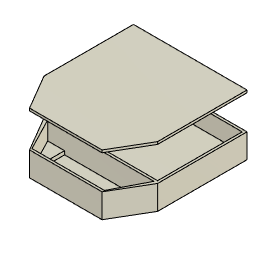
mainboard v1 (Autodesk Fusion 360 design; units mm, degrees)
Autodesk Fusion 360 part; units mm, degrees
sketch "Sketch1" plane through (0, 0, 0) normal (0, 0, 1) x (1, 0, 0)
  line L0 (0, 0) -> (90, 0)
  line L1 (90, 0) -> (90, 70)
  line L2 (90, 70) -> (0, 70)
  line L3 (0, 70) -> (0, 0)
  circle A0 centre (86, 65) radius 1.5
  circle A1 centre (4, 65) radius 1.5
  circle A2 centre (4, 5) radius 1.5
  circle A3 centre (86, 5) radius 1.5
  line L4 (15, -1) -> (75, -1)
  line L5 (75, -1) -> (75, -29)
  line L6 (75, -29) -> (15, -29)
  line L7 (15, -29) -> (15, -1)
  line L8 (0, 0) -> (15, -29)
  line L9 (90, 0) -> (75, -29)
  line L10 (92, -2) -> (92, 72)
  line L11 (92, 72) -> (-2, 72)
  line L12 (-2, 72) -> (-2, -2)
  line L13 (-2, -2) -> (92, -2)
  line L14 (75, -31) -> (15, -31)
  line L15 (75, -31) -> (92, -2)
  line L16 (15, -31) -> (-2, -2)
  dimension "d1" = 90
  dimension "d2" = 70
  dimension "d3" = 3
  dimension "d4" = 3
  dimension "d5" = 3
  dimension "d6" = 3
  dimension "d7" = 4
  dimension "d8" = 4
  dimension "d9" = 4
  dimension "d10" = 4
  dimension "d11" = 5
  dimension "d12" = 5
  dimension "d13" = 5
  dimension "d14" = 5
  dimension "d15" = 60
  dimension "d16" = 28
  dimension "d17" = 15
  dimension "d19" = 1
  dimension "d20" = 2
  dimension "d21" = -2
  constraint horizontal L0
  constraint vertical L1
  constraint horizontal L2
  constraint vertical L3
  constraint coincident L0.start L3.end
  constraint horizontal L4
  constraint vertical L5
  constraint horizontal L6
  constraint vertical L7
  measures "d1" distance of L0.start L0.end
  measures "d2" distance of L0.start L2.end
  measures "d3" diameter of A0
  measures "d4" diameter of A1
  measures "d5" diameter of A2
  measures "d6" diameter of A3
  measures "d7" distance of L3 A1.centre
  measures "d8" distance of L3 A2.centre
  measures "d9" distance of L1 A0.centre
  measures "d10" distance of L1 A3.centre
  measures "d11" distance of L2 A1.centre
  measures "d12" distance of L2 A0.centre
  measures "d13" distance of L0 A3.centre
  measures "d14" distance of L0 A2.centre
  measures "d15" distance of L4.start L4.end
  measures "d16" distance of L4.start L6.end
  measures "d17" distance of L3 L7
  measures "d19" distance of L0 L4
extrude "Extrude1" add sketch "Sketch1" along normal blind 5 contours L0 L1 L2 L3 makes body 1
extrude "Extrude2" add sketch "Sketch1" along normal blind 5 contours L1 L2 L3 L8 L9 L10 L11 L12 L13 | L0 L4 L5 L7 L8 L9 L13 | L7 L8 L13 | L6 L8 L9 L13 L14 L15 L16 | L5 L9 L13 bodies 1
extrude "Extrude3" add sketch "Sketch1" along normal blind 2 contours L5 L6 L7 L13 bodies 1
extrude "Extrude4" add sketch "Sketch1" along normal blind 20 contours L1 L2 L3 L8 L9 L10 L11 L12 L13 bodies 1
extrude "Extrude5" add sketch "Sketch1" along normal blind 20 contours L0 L4 L5 L7 L8 L9 L13 | L6 L8 L9 L13 L14 L15 L16 | L4 L5 L7 L13 bodies 1
extrude "Extrude6" add sketch "Sketch1" against normal blind 2 separate body contours L0 L1 L2 L3 | L1 L2 L3 L8 L9 L10 L11 L12 L13 | L0 L4 L5 L7 L8 L9 L13 | L7 L8 L13 | L6 L8 L9 L13 L14 L15 L16 | L5 L9 L13 | L5 L6 L7 L13 | L4 L5 L7 L13 | A0 | A1 | A2 | A3 makes body 2
move_body "Move1" bodies 2 to x (1, 0, 0) y (0, 1, 0) z (0, 0, 1) at (0, 0, 50)
